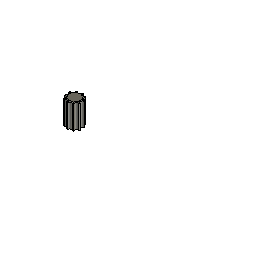
Dial (Autodesk Fusion 360 design; units mm, degrees)
Autodesk Fusion 360 part; units mm, degrees
sketch "Sketch1" plane through (0, 0, 103) normal (0, 0, 1) x (-1, 0, 0)
  line L0 (15.5, 13) -> (15.5, -13)
  line L1 (15.5, -13) -> (60, -13)
  line L2 (60, -13) -> (60, 13)
  line L3 (60, 13) -> (15.5, 13)
  circle A0 centre (23, -4) radius 3.5
  line L4 (34.2035, 8.9925) -> (52.2035, 8.9925)
  arc A1 (52.2035, 5.9925) -> (52.2035, 8.9925) centre (52.2035, 7.4925) ccw
  line L5 (52.2035, 5.9925) -> (34.2035, 5.9925)
  arc A2 (34.2035, 8.9925) -> (34.2035, 5.9925) centre (34.2035, 7.4925) ccw
  line L6 (19.9444, 9.4997) -> (28.9444, 9.4997)
  line L7 (28.9444, 9.4997) -> (28.9444, 5.4997)
  line L8 (28.9444, 5.4997) -> (19.9444, 5.4997)
  line L9 (19.9444, 5.4997) -> (19.9444, 9.4997)
  circle A3 centre (50.1476, -3.0488) radius 6
  circle A4 centre (50.1476, -3.0488) radius 6.5
  circle A5 centre (43.6476, -3.0488) radius 1.5
  circle A6 centre (44.889, -6.8694) radius 1.5
  circle A7 centre (48.139, -9.2306) radius 1.5
  circle A8 centre (52.1562, -9.2306) radius 1.5
  circle A9 centre (55.4062, -6.8694) radius 1.5
  circle A10 centre (56.6476, -3.0488) radius 1.5
  circle A11 centre (55.4062, 0.7719) radius 1.5
  circle A12 centre (52.1562, 3.1331) radius 1.5
  circle A13 centre (48.139, 3.1331) radius 1.5
  circle A14 centre (44.889, 0.7719) radius 1.5
  dimension "d128" = 13
  dimension "d129" = 3
  dimension "d131" = 360
  constraint concentric A3 A4
  constraint coincident A4 A5.centre
  measures "d128" diameter of A4
  measures "d129" diameter of A5
extrude "Extrude1" add sketch "Sketch1" along normal blind 20 contours A3 A5 A6 A7 A8 A9 A10 A11 A12 A13 A14 | A3 A4 A10 A11 | A3 A4 A9 A10 | A3 A4 A11 A12 | A3 A4 A8 A9 | A3 A4 A12 A13 | A3 A4 A7 A8 | A3 A4 A13 A14 | A3 A4 A6 A7 | A3 A4 A5 A14 | A3 A4 A5 A6
fillet "Fillet1" radius 0.5 9 edges at (-54.1927, 5.9877, 123) (-56.3295, 5.0574, 123) (-55.1476, 3.0488, 123) (-56.3295, 1.0401, 123) (-54.1927, 0.1098, 123) (-51.6927, -1.7065, 123) (-53.9682, -2.2099, 123) (-50.1476, -3.4512, 123) (-48.6025, -1.7065, 123) 1 faces at (-51.5204, 4.0363, 123)
